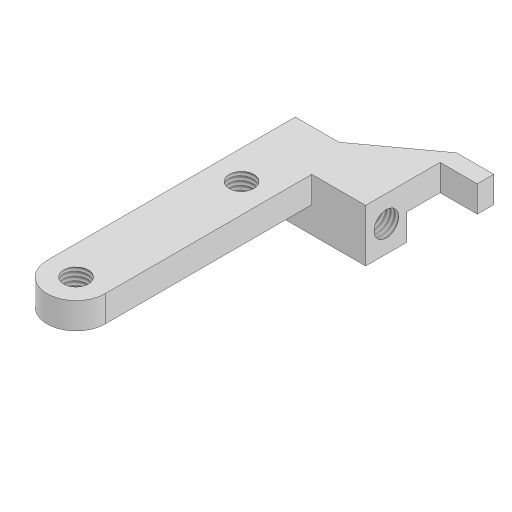
# Autodesk Inventor part: mgn9SlideBearingHolder
Saved by Autodesk Inventor 2023 (Build 270158000, 158)
## iProperties
Created: 2022-11-03
Part Number: mgn9SlideBearingHolder
Material: Generic
Document SubType Name: Modeling
Designer: deli
Density: 1 g/cm^3
Appearance: Default
Mass: 1.0508 g
Surface Area: 11.5801 cm^2
Volume: 1.0508 cm^3
Author: deli
Autodesk Inventor part; units mm, degrees
ref_plane "YZ Plane" through (0, 0, 0) normal (1, 0, 0) x (0, 1, 0)
ref_plane "XZ Plane" through (0, 0, 0) normal (0, 1, 0) x (-1, 0, 0)
ref_plane "XY Plane" through (0, 0, 0) normal (0, 0, 1) x (1, 0, 0)
sketch "Sketch1" plane through (0, 0, 0) normal (0, 1, 0) x (-1, 0, 0)
  circle A0 centre (7.2873, 50.1345) radius 1.5
  circle A1 centre (7.2873, 30.1345) radius 1.5
  arc A2 (10.7873, 50.1345) -> (3.7873, 50.1345) centre (7.2873, 50.1345) ccw
  line L0 (10.7873, 50.1345) -> (10.7873, 23.9862)
  line L1 (3.7873, 25.1345) -> (3.7873, 50.1345)
  line L2 (-2.7127, 16.1345) -> (-2.7127, 25.1345)
  line L3 (-2.7127, 25.1345) -> (3.7873, 25.1345)
  line L4 (10.7873, 23.9862) -> (-2.7127, 14.1345)
  line L5 (-2.7127, 14.1345) -> (-7.2127, 14.1345)
  line L6 (-7.2127, 14.1345) -> (-7.2127, 16.1345)
  line L7 (-2.7127, 16.1345) -> (-7.2127, 16.1345)
  point P0 (0, 0)
  dimension "d0" = 3
  dimension "d1" = 2
  dimension "d2" = 20
  dimension "d20" = 10
  dimension "d27" = 3.5
  dimension "d28" = 5
  dimension "d30" = 9
  dimension "d31" = 2
  dimension "d35" = 4.5
  constraints: 16 end point, 3 centre point, 2 horizontal, 2 perpendicular, 2 point on circle, 2 tangent, 1 coincident, 1 equal radius, 1 parallel, 1 vertical
  measures "d0" diameter of A0
  measures "d1" radial gap between concentric circles of A2 A0
  measures "d2" distance of A0.centre A1.centre
  measures "d20" distance from line of A1.centre L2
  measures "d27" distance from line of L0 A1.centre
  measures "d28" distance from line of L3 A1.centre
  measures "d30" distance of L2.start L2.end
  measures "d31" distance of L5.end L6.end
  measures "d35" distance of L2.start L6.end
extrude "Extrusion1" add sketch "Sketch1" along normal blind 3.175
sketch "Sketch2" plane through (0, 3.175, 0) normal (0, 1, 0) x (1, 0, 0)
  line L0 (-10.7873, -20.1345) -> (2.7127, -20.1345)
  line L1 (2.7127, -20.1345) -> (2.7127, -25.1345)
  line L2 (2.7127, -25.1345) -> (-10.7873, -25.1345)
  line L3 (-10.7873, -25.1345) -> (-10.7873, -20.1345)
  point P0 (0, 0)
  point P1 (2.7127, -25.1345)
  constraints: 8 end point, 2 coincident, 2 parallel, 1 horizontal, 1 perpendicular
extrude "Extrusion2" add sketch "Sketch2" against normal blind 6.35
thread "Thread1" size "M3x0.5" class "6H" standard "ANSI Metric M Profile" full length
thread "Thread3" size "M3x0.5" class "6H" standard "ANSI Metric M Profile" full length
sketch "Sketch4" plane through (2.7127, 0, 25.1345) normal (1, 0, 0) x (0, 0, -1)
  circle A0 centre (2.5, 0) radius 1.5
  line L0 (0, -3.175) -> (0, 3.175) projected
  line L1 (0, 3.175) -> (9, 3.175) projected
  point P0 (25.1345, 0)
  dimension "d32" = 3
  dimension "d33" = 1
  dimension "d34" = 3.175
  constraints: 1 centre point
  measures "d32" diameter of A0
  measures "d33" distance edge to line of A0 L0
  measures "d34" distance from line of L1 A0.centre
extrude "Extrusion4" cut sketch "Sketch4" against normal blind 8
thread "Thread4" size "M3x0.5" class "6H" standard "ANSI Metric M Profile" full length
equation "\"d27\" = d1 + 0.5 * d0"
body "Solid1"
